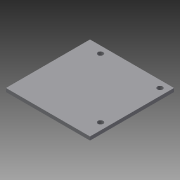
# Autodesk Inventor part: contorller kort
Saved by Autodesk Inventor 2015 (Build 190159000, 159)
## iProperties
Created: 2015-08-04
Part Number: contorller kort
Material: Generic
Document SubType Name: Modeling
Designer: Simen
Density: 1 g/cm^3
Appearance: Default
Author: Simen
Autodesk Inventor part; units mm, degrees
ref_plane "YZ Plane" through (0, 0, 0) normal (1, 0, 0) x (0, 1, 0)
ref_plane "XZ Plane" through (0, 0, 0) normal (0, 1, 0) x (-1, 0, 0)
ref_plane "XY Plane" through (0, 0, 0) normal (0, 0, 1) x (1, 0, 0)
sketch "Sketch1" plane through (0, 0, 0) normal (0, 0, 1) x (1, 0, 0)
  line L0 (5.5291, -4.6499) -> (-42.4709, -4.6499)
  line L1 (-42.4709, -4.6499) -> (-42.4709, -52.6499)
  line L2 (-42.4709, -52.6499) -> (5.5291, -52.6499)
  line L3 (5.5291, -52.6499) -> (5.5291, -4.6499)
  line L4 (5.5291, -4.6499) -> (5.5291, -8.6499)
  line L5 (5.5291, -8.6499) -> (1.5291, -8.6499)
  circle A0 centre (1.5291, -8.6499) radius 1.5
  line L6 (-42.4709, -4.6499) -> (-42.4709, -8.6499)
  line L7 (-42.4709, -8.6499) -> (-32.4709, -8.6499)
  circle A1 centre (-32.4709, -8.6499) radius 1.5
  line L8 (5.5291, -52.6499) -> (5.5291, -42.6499)
  line L9 (5.5291, -42.6499) -> (1.5291, -42.6499)
  circle A2 centre (1.5291, -42.6499) radius 1.5
  point P0 (0, 0)
  dimension "d0" = 48
  dimension "d1" = 48
  dimension "d2" = 4
  dimension "d3" = 4
  dimension "d4" = 3
  dimension "d5" = 4
  dimension "d6" = 10
  dimension "d7" = 3
  dimension "d8" = 10
  dimension "d9" = 4
  dimension "d10" = 3
  constraints: 20 end point, 3 centre point, 3 coincident, 3 perpendicular, 3 point on line, 2 horizontal, 2 parallel
  measures "d0" distance of L2.end L1.end
  measures "d1" distance of L1.end L0.end
  measures "d2" distance of L0.start L4.end
  measures "d3" distance of L4.end L5.end
  measures "d4" diameter of A0
  measures "d5" distance of L0.end L6.end
  measures "d6" distance of L6.end L7.end
  measures "d7" diameter of A1
  measures "d8" distance of L2.end L8.end
  measures "d9" distance of L8.end L9.end
  measures "d10" diameter of A2
extrude "Extrusion1" add sketch "Sketch1" along normal blind 2
body "Solid1"
